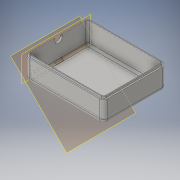
# Autodesk Inventor part: RFID_Box
Saved by Autodesk Inventor 2016 (Build 200138000, 138)
## iProperties
Created: 2015-09-30
Part Number: RFID_Box
Material: Generic
Document SubType Name: Modeling
Designer: Drew
Density: 1 g/cm^3
Appearance: Default
Author: Drew
Autodesk Inventor part; units mm, degrees
ref_plane "YZ Plane" through (0, 0, 0) normal (1, 0, 0) x (0, 1, 0)
ref_plane "XZ Plane" through (0, 0, 0) normal (0, 1, 0) x (-1, 0, 0)
ref_plane "XY Plane" through (0, 0, 0) normal (0, 0, 1) x (1, 0, 0)
sketch "Sketch1" plane through (0, 0, 0) normal (0, 1, 0) x (-1, 0, 0)
  line L0 (2.728, 3.799) -> (-60.772, 3.799)
  line L1 (-60.772, 3.799) -> (-60.772, -47.001)
  line L2 (-60.772, -47.001) -> (2.728, -47.001)
  line L3 (2.728, -47.001) -> (2.728, 3.799)
  dimension "d0" = 63.5
  dimension "d1" = 50.8
  constraints: 8 end point, 2 parallel, 1 horizontal, 1 perpendicular
  measures "d0" distance of L2.end L1.end
  measures "d1" distance of L1.end L0.end
extrude "Extrusion1" add sketch "Sketch1" along normal blind 1.5875
sketch "Sketch2" plane through (0, 1.5875, 0) normal (0, 1, 0) x (1, 0, 0)
  line L0 (59.1845, 45.4135) -> (-1.1405, 45.4135)
  line L1 (-1.1405, 45.4135) -> (-1.1405, -2.2115)
  line L2 (-1.1405, -2.2115) -> (59.1845, -2.2115)
  line L3 (59.1845, -2.2115) -> (59.1845, 45.4135)
  line L4 (60.772, 47.001) -> (-2.728, 47.001) projected
  line L5 (-2.728, 47.001) -> (-2.728, -3.799) projected
  line L6 (60.772, -3.799) -> (60.772, 47.001) projected
  line L7 (-2.728, -3.799) -> (60.772, -3.799) projected
  point P0 (0, 0)
  dimension "d4" = 1.5875
  dimension "d5" = 1.5875
  dimension "d6" = 1.5875
  dimension "d7" = 1.5875
  constraints: 8 end point, 2 parallel, 1 horizontal, 1 perpendicular
  measures "d4" distance from line of L4 L0.end
  measures "d5" distance from line of L5 L1.end
  measures "d6" distance from line of L6 L2.end
  measures "d7" distance from line of L7 L2.end
extrude "Extrusion2" add sketch "Sketch2" along normal blind 17.4625
fillet "Fillet1" radius 3.302 8 edges at (29.022, 0, 3.799) (60.772, 0, -21.601) (29.022, 0, -47.001) (-2.728, 0, -21.601) (60.772, 9.525, -47.001) (60.772, 9.525, 3.799) (-2.728, 9.525, 3.799) (-2.728, 9.525, -47.001)
fillet "Fillet2" radius 1.5875 8 edges at (-1.1405, 10.3188, -45.4135) (29.022, 1.5875, -45.4135) (-1.1405, 1.5875, -21.601) (-1.1405, 10.3188, 2.2115) (29.022, 1.5875, 2.2115) (59.1845, 10.3188, 2.2115) (59.1845, 1.5875, -21.601) (59.1845, 10.3188, -45.4135)
sketch "Sketch4" plane through (0, 19.05, 0) normal (0, 1, 0) x (1, 0, 0)
  line L0 (0.447, 45.4135) -> (57.597, 45.4135) projected
  arc A0 (0.447, 45.4135) -> (-1.1405, 43.826) centre (0.447, 43.826) ccw projected
  line L1 (-1.1405, -0.624) -> (-1.1405, 43.826) projected
  arc A1 (59.1845, 43.826) -> (57.597, 45.4135) centre (57.597, 43.826) ccw projected
  line L2 (59.1845, 43.826) -> (59.1845, -0.624) projected
  arc A2 (57.597, -2.2115) -> (59.1845, -0.624) centre (57.597, -0.624) ccw projected
  line L3 (57.597, -2.2115) -> (0.447, -2.2115) projected
  arc A3 (-1.1405, -0.624) -> (0.447, -2.2115) centre (0.447, -0.624) ccw projected
  line L4 (0.2977, 46.0073) -> (57.7462, 46.0073)
  line L5 (59.7782, 43.9753) -> (59.7782, -0.7732)
  line L6 (57.7462, -2.8052) -> (0.2977, -2.8052)
  line L7 (-1.7343, -0.7732) -> (-1.7343, 43.9753)
  line L8 (57.47, 47.001) -> (0.574, 47.001) projected
  line L9 (-2.728, 43.699) -> (-2.728, -0.497) projected
  arc A4 (0.574, 47.001) -> (-2.728, 43.699) centre (0.574, 43.699) ccw projected
  arc A5 (60.772, 43.699) -> (57.47, 47.001) centre (57.47, 43.699) ccw projected
  line L10 (60.772, -0.497) -> (60.772, 43.699) projected
  arc A6 (57.47, -3.799) -> (60.772, -0.497) centre (57.47, -0.497) ccw projected
  line L11 (0.574, -3.799) -> (57.47, -3.799) projected
  arc A7 (-2.728, -0.497) -> (0.574, -3.799) centre (0.574, -0.497) ccw projected
  line L12 (9.3601, 46.0073) -> (9.3601, 47.001)
  line L13 (9.9735, 46.0073) -> (9.9735, 45.2135)
  line L14 (-1.7343, 35.9118) -> (-2.728, 35.9118)
  line L15 (-1.7343, 35.9118) -> (-1.1405, 35.9118)
  line L16 (3.5402, -2.2115) -> (3.5402, -2.8052)
  line L17 (3.9514, -2.8052) -> (3.9514, -3.799)
  line L18 (59.1845, 4.7048) -> (59.7782, 4.7048)
  line L19 (59.7782, 4.7048) -> (60.772, 4.7048)
  arc A8 (0.2977, 46.0073) -> (-1.7343, 43.9753) centre (0.2977, 43.9753) ccw
  arc A9 (59.7782, 43.9753) -> (57.7462, 46.0073) centre (57.7462, 43.9753) ccw
  arc A10 (-1.7343, -0.7732) -> (0.2977, -2.8052) centre (0.2977, -0.7732) ccw
  arc A11 (57.7462, -2.8052) -> (59.7782, -0.7732) centre (57.7462, -0.7732) ccw
  point P0 (0, 0)
  dimension "d20" = 2.032
  dimension "d21" = 2.032
  dimension "d22" = 2.032
  dimension "d23" = 2.032
  dimension "d26" = 0.9938
  dimension "d27" = 0.9938
  dimension "d28" = 0.9938
  dimension "d29" = 0.9938
  constraints: 24 end point, 15 point on line, 8 point on circle, 8 tangent, 5 perpendicular, 4 centre point, 2 parallel, 1 horizontal
  measures "d20" radius of A8
  measures "d21" radius of A9
  measures "d22" radius of A10
  measures "d23" radius of A11
  measures "d26" distance of L17.start L17.end
  measures "d27" distance of L14.start L14.end
  measures "d28" distance of L12.start L12.end
  measures "d29" distance of L18.end L19.end
extrude "Extrusion4" cut sketch "Sketch4" against normal blind 1.5875 contours L4 L12 L8 A5 L10 L19 L5 A9 | L4 A8 L7 L14 L9 A4 L8 L12 | L7 A10 L6 L17 L11 A7 L9 L14 | L19 L10 A6 L11 L17 L6 A11 L5
ref_plane "Work Plane1" through (-1.1405, 3.175, -33.5073) normal (0.7071, 0.7071, 0) x (0, 0, 1)
sketch "Sketch8" plane through (-1.1405, 3.175, -33.5073) normal (0.7071, 0.7071, 0) x (0, 0, 1)
  line L0 (34.1313, 0) -> (34.1313, 2.2451) projected
  line L1 (-10.3187, 0) -> (34.1313, 0) projected
  line L2 (34.1313, 2.2451) -> (-10.3187, 2.2451) projected
  line L3 (-10.3187, 2.2451) -> (-10.3187, 0) projected
  line L4 (14.9063, -0.1275) -> (8.9063, -0.1275)
  line L5 (8.9063, -0.1275) -> (8.9063, 2.3725)
  line L6 (8.9063, 2.3725) -> (14.9063, 2.3725)
  line L7 (14.9063, 2.3725) -> (14.9063, -0.1275)
  line L8 (14.9063, 1.1225) -> (34.1313, 1.1225)
  line L9 (8.9063, 1.8195) -> (-10.3187, 1.8195)
  line L10 (14.1632, 0) -> (14.1632, -0.1275)
  line L11 (13.7933, 2.3725) -> (13.7933, 2.2451)
  point P0 (33.5073, 3.0515)
  dimension "d43" = 6
  dimension "d44" = 2.5
  constraints: 16 end point, 6 point on line, 5 perpendicular, 4 parallel, 2 midpoint, 1 horizontal
  measures "d43" distance of L5.end L6.end
  measures "d44" distance of L4.end L5.end
extrude "Extrusion7" cut sketch "Sketch8" against normal blind 1.4 contours L7 L4 L10 L1 | L1 L5 L2 L7 | L10 L4 L5 L1 | L2 L11 L6 L7 | L2 L5 L6 L11
ref_plane "Work Plane2" through (-2.728, 3.302, -34.301) normal (1, 0, 0) x (0, 0, -1)
sketch "Sketch9" plane through (-2.728, 3.302, -34.301) normal (1, 0, 0) x (0, 0, -1)
  line L0 (-34.798, 14.1605) -> (9.398, 14.1605) projected
  line L1 (12.7, 14.1605) -> (12.7, 0) projected
  line L2 (-38.1, 0) -> (-38.1, 14.1605) projected
  circle A0 centre (-12.7, 14.1605) radius 3
  line L3 (-12.7, 14.1605) -> (12.7, 14.1605)
  line L4 (12.7, 0) -> (12.7, 14.1605) projected
  line L5 (-12.7, 14.1605) -> (-38.1, 14.1605)
  line L6 (-38.1, 14.1605) -> (-38.1, 0) projected
  line L7 (9.398, 14.1605) -> (-34.798, 14.1605) projected
  line L8 (-9.7, 14.1605) -> (-9.7, 15.748)
  line L9 (-34.925, 15.748) -> (9.525, 15.748) projected
  line L10 (-15.7, 14.1605) -> (-15.7, 15.748)
  point P0 (-34.301, -3.302)
  dimension "d47" = 6
  constraints: 8 end point, 7 point on line, 2 collinear, 2 point on circle, 1 centre point, 1 parallel, 1 perpendicular, 1 tangent, 1 vertical
  measures "d47" diameter of A0
extrude "Extrusion9" cut sketch "Sketch9" along normal blind 3
equation "\"d5\" = d4"
equation "\"d6\" = d4"
equation "\"d7\" = d4"
body "Solid1"
